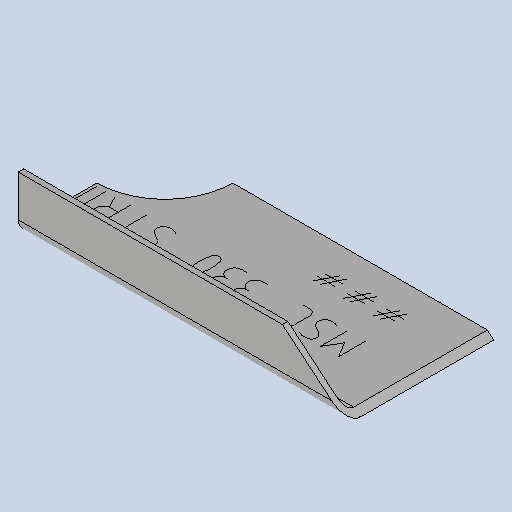
# Autodesk Inventor part: MSC 330 STRINGER BOARD  ###
Saved by Autodesk Inventor 2025.1 (Build 291241020, 241B)
## iProperties
Created: 2024-04-28
Part Number: MSC 330 STRINGER BOARD  ###
Material: Stainless Steel
Document SubType Name: Sheet Metal
Designer: pokla
Stock Number: MSC 324 стрингер борт ###
Mass: 87.4423 g
Surface Area: 116.196 cm^2
Volume: 10.9303 cm^3
Density: 8 g/cm^3
Flat Pattern Width: 7.0202 cm
Flat Pattern Length: 12.1125 cm
Flat Pattern Area: 85.0324 cm^2
Sheet Metal Rule: AISI304 2mm Die16
Sheet Metal Width: 70.202 mm
Sheet Metal Length: 121.125 mm
Sheet Metal Area: 8503.238 mm^2
Appearance: Default
Author: admin
Autodesk Inventor part; units mm, degrees
ref_plane "YZ Plane" through (0, 0, 0) normal (1, 0, 0) x (0, 1, 0)
ref_plane "XZ Plane" through (0, 0, 0) normal (0, 1, 0) x (-1, 0, 0)
ref_plane "XY Plane" through (0, 0, 0) normal (0, 0, 1) x (1, 0, 0)
sketch "Sketch1" plane through (0, 0, 0) normal (0, 0, 1) x (1, 0, 0)
  line L0 (-490, 54) -> (490, 54)
  line L1 (490, 54) -> (490, 0)
  line L2 (490, 0) -> (-490, 0)
  line L3 (-490, 0) -> (-490, 54)
  point P0 (0, 0)
  point P1 (0, 0)
  dimension "d0" = 980
  dimension "d1" = 54
  measures "d0" distance of L1.end L2.end
  measures "d1" distance of L0.end L1.end
extrude "Plate1" add sketch "Sketch1" along normal blind 2
sketch "Sketch2" plane through (490, 2, 0) normal (0, -1, 0) x (1, 0, 0)
  line L0 (-980, 0) -> (0, 0)
  line L1 (0, 0) -> (0, 20)
  line L2 (0, 20) -> (-980, 20)
  line L3 (-980, 20) -> (-980, 0)
  constraints: 6 end point, 1 horizontal, 1 perpendicular, 1 vertical
edge flange "Flange1" height 20 angle 90 thickness 2 bend radius 2.75 thickness toward (0, -1, 0) relief round relief width 2 relief depth 1 edges at (0, 0, 2) wall of the first edge with corners at (-490, 2, 0) (490, 2, 0) (490, 2, 20) (-490, 2, 20)
bend "Bend1"
corner "Corner1"
sketch "Sketch5" plane through (0, 0, 0) normal (0, 0, -1) x (-1, 0, 0)
  line L0 (490, 54) -> (-490, 54) projected
  line L1 (490, 0) -> (-490, 0) projected
  circle A0 centre (0, 54) radius 25
  line L2 (243.95, 54) -> (246.05, 54)
  line L3 (246.05, 54) -> (246.05, 29)
  line L4 (246.05, 29) -> (243.95, 29)
  line L5 (243.95, 29) -> (243.95, 54)
  line L6 (-243.95, 54) -> (-246.05, 54)
  line L7 (-246.05, 54) -> (-246.05, 29)
  line L8 (-246.05, 29) -> (-243.95, 29)
  line L9 (-243.95, 29) -> (-243.95, 54)
  line L10 (0, 54) -> (0, 0) construction
  circle A1 centre (490, 54) radius 25
  point P0 (0, 0)
  point P1 (245, 29)
  point P2 (-245, 29)
  point P3 (246.05, 54)
  point P4 (-25, 54)
  point P5 (25, 54)
  point P6 (-246.05, 54)
  dimension "d45" = 50
  dimension "d48" = 2.1
  dimension "d49" = 490
  dimension "d51" = 29
  dimension "d52" = 25
  constraints: 18 end point, 4 midpoint, 4 parallel, 3 perpendicular, 2 centre point, 2 collinear, 2 horizontal, 2 point on line, 1 coincident, 1 equal radius, 1 other
  measures "d45" diameter of A0
  measures "d48" distance of L7.end L8.end
  measures "d49" distance of point (245, 29) point (-245, 29)
  measures "d51" distance between parallel lines of L8 L1
  measures "d52" distance between parallel lines of L0 L8
extrude "Extrusion1" cut sketch "Sketch5" against normal through all contours L3 L4 L5 L0 | L9 L8 L7 L0 | A1
sketch "Sketch9" plane through (0, 0, 2) normal (0, 0, 1) x (1, 0, 0)
  line L0 (-389.1031, 29.596) -> (-389.1031, 17.596) construction
  line L1 (-389.1031, 17.596) -> (-589.1031, 17.596) construction
  line L2 (-589.1031, 17.596) -> (-589.1031, 29.596) construction
  line L3 (-589.1031, 29.596) -> (-389.1031, 29.596) construction
  line L4 (-490, 54) -> (490, 54) projected
  point P0 (0, 0)
  point P1 (1.05, 68)
  point P2 (490, 54)
  dimension "d40" = 200
  dimension "d41" = 12
  constraints: 1 horizontal, 3 other
  measures "d40" distance of L0.end L1.end
  measures "d41" distance of L1.end L2.end
mark "Mark2"
sketch "Sketch10" plane through (-490, 0, 20) normal (0, -1, 0) x (1, 0, 0)
  line L0 (980, -20) -> (736.05, -20) projected
  line L1 (0, 0) -> (980, 0) projected
  line L2 (980, -20) -> (97.2902, -20)
  line L3 (97.2902, -20) -> (97.2902, 0)
  line L4 (97.2902, 0) -> (980, 0)
  line L5 (980, 0) -> (980, -20)
  line L6 (97.2902, 0) -> (121.1253, -20)
  point P0 (490, -20)
  point P1 (736.05, -20)
  dimension "d53" = 882.7098
  dimension "d54" = 50
  constraints: 10 end point, 2 parallel, 2 point on line, 1 horizontal, 1 perpendicular
  measures "d53" distance between parallel lines of L5 L3
  measures "d54" angle of L6 L3
extrude "Extrusion4" cut sketch "Sketch10" against normal through all contours L0 L2 L6 L1 L5
equation "\"d2\" = Thickness"
equation "\"d3\" = BendReliefWidth"
equation "\"d4\" = BendReliefDepth"
equation "\"d5\" = MinimumRemnant"
equation "\"d6\" = TransitionRadius"
equation "\"d9\" = BendRadius"
equation "\"d10\" = CornerReliefSize"
equation "\"d11\" = GapSize"
equation "\"d12\" = JacobiRadiusSize"
equation "\"BendReliefWidth\" = Thickness"
equation "\"BendReliefDepth\" = 0.5 * Thickness"
equation "\"CornerReliefSize\" = 4 * Thickness"
equation "\"MinimumRemnant\" = 2 * Thickness"
equation "\"TransitionRadius\" = BendRadius"
equation "\"JacobiRadiusSize\" = BendRadius"
equation "\"GapSize\" = Thickness"
equation "\"Thickness\" = 2"
equation "\"BendRadius\" = 2.75"
body "Solid1"
